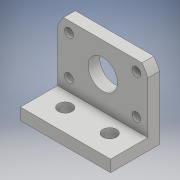
# Autodesk Inventor part: X-axis Ball Screw Support
Saved by Autodesk Inventor 2018 (Build 220112000, 112)
## iProperties
Created: 2018-03-20
Part Number: X-axis Ball Screw Support
Material: Generic
Document SubType Name: Modeling
Designer: M201291
Density: 1 g/cm^3
Appearance: Default
Author: M201291
Autodesk Inventor part; units mm, degrees
ref_plane "YZ Plane" through (0, 0, 0) normal (1, 0, 0) x (0, 1, 0)
ref_plane "XZ Plane" through (0, 0, 0) normal (0, 1, 0) x (-1, 0, 0)
ref_plane "XY Plane" through (0, 0, 0) normal (0, 0, 1) x (1, 0, 0)
sketch "Sketch1" plane through (0, 0, 0) normal (0, 0, 1) x (1, 0, 0)
  line L0 (0, 0) -> (46, 0)
  line L1 (46, 0) -> (46, -25)
  line L2 (46, -25) -> (0, -25)
  line L3 (0, -25) -> (0, 0)
  dimension "d0" = 46
  dimension "d1" = 25
  constraints: 8 end point, 2 parallel, 1 horizontal, 1 perpendicular
  measures "d0" distance of L1.end L2.end
  measures "d1" distance of L0.end L1.end
extrude "Extrusion1" add sketch "Sketch1" along normal blind 6
sketch "Sketch2" plane through (0, 0, 6) normal (0, 0, 1) x (1, 0, 0)
  line L0 (46, 0) -> (0, 0) construction
  line L1 (23, 0) -> (23, -25) construction
  line L2 (0, -25) -> (46, -25) construction
  line L3 (0, 0) -> (0, -25) construction
  line L4 (0, -13.8) -> (11.65, -13.8) construction
  point P0 (34.35, -13.8)
  dimension "d5" = 13.8
  dimension "d34" = 11.65
  constraints: 4 end point, 2 midpoint, 1 coincident, 1 horizontal, 1 point on line, 1 symmetric about line
  measures "d5" distance from line of L0 L4.end
  measures "d34" distance of L4.start L4.end
hole "Hole1" at (11.65, -13.8, 6) at (34.35, -13.8, 6) direction (0, 0, -1) diameter 7 end through all
sketch "Sketch3" plane through (0, 0, 6) normal (0, 0, 1) x (1, 0, 0)
  line L0 (46, -25) -> (46, 0) projected
  line L1 (0, 0) -> (46, 0)
  line L2 (46, 0) -> (46, -6)
  line L3 (46, -6) -> (0, -6)
  line L4 (0, -6) -> (0, 0)
  dimension "d13" = 6
  constraints: 8 end point, 2 parallel, 1 horizontal, 1 perpendicular, 1 point on line
  measures "d13" distance of L1.end L2.end
extrude "Extrusion2" add sketch "Sketch3" along normal blind 31.55
sketch "Sketch4" plane through (0, 0, 0) normal (0, 1, 0) x (1, 0, 0)
  line L0 (0, 0) -> (0, -37.55) construction
  line L1 (0, -12.254) -> (5.824, -12.254) construction
  line L2 (0, -6) -> (46, -6) construction
  line L3 (0, 0) -> (46, 0) construction
  line L4 (23, 0) -> (23, -37.55) construction
  line L5 (46, -37.55) -> (0, -37.55) construction
  line L6 (0, -32.254) -> (5.824, -32.254) construction
  point P0 (40.176, -32.254)
  point P1 (40.176, -12.254)
  dimension "d16" = 12.254
  dimension "d17" = 5.824
  dimension "d18" = 20
  constraints: 6 end point, 2 coincident, 2 midpoint, 2 point on line, 2 symmetric about line, 1 horizontal, 1 parallel
  measures "d16" distance between parallel lines of L3 L1
  measures "d17" distance of L1.start L1.end
  measures "d18" distance between parallel lines of L1 L6
hole "Hole2" at (5.824, 0, 32.254) at (5.824, 0, 12.254) at (40.176, 0, 32.254) at (40.176, 0, 12.254) direction (0, -1, 0) diameter 4.5 end through all
sketch "Sketch5" plane through (0, -6, 6) normal (0, -1, 0) x (1, 0, 0)
  line L0 (0, 31.55) -> (46, 31.55) projected
  point P0 (0, -6)
  point P1 (23, 16.55)
  dimension "d26" = 15
  measures "d26" distance from line of L0 point (23, 16.55)
hole "Hole3" at (23, -6, 22.55) direction (0, 1, 0) diameter 15 end through all
sketch "Sketch6" plane through (0, 0, 0) normal (0, 1, 0) x (1, 0, 0)
  circle A0 centre (23, -22.55) radius 7.5 projected
  line L0 (0, -37.55) -> (46, -37.55) construction
  line L1 (46, -37.55) -> (0, -37.55) construction
  line L2 (0, -37.55) -> (0, -27.1443) construction
  line L3 (0, 0) -> (0, -37.55) construction
  line L4 (46, -37.55) -> (46, -28.4346) construction
  line L5 (46, -6) -> (46, -37.55) construction
  arc A1 (0, -32.348) -> (3, -37.55) centre (23, -22.55) ccw
  arc A2 (43, -37.55) -> (46, -32.348) centre (23, -22.55) ccw
  line L6 (43, -37.55) -> (46, -37.55)
  line L7 (3, -37.55) -> (0, -37.55)
  line L8 (0, -32.348) -> (0, -37.55)
  line L9 (46, -37.55) -> (46, -32.348)
  constraints: 14 end point, 6 point on line, 5 collinear, 4 point on circle, 2 centre point, 1 coincident
extrude "Extrusion3" cut sketch "Sketch6" against normal up to next contours A1 L7 L8 | A2 L9 L6
body "Solid1"
